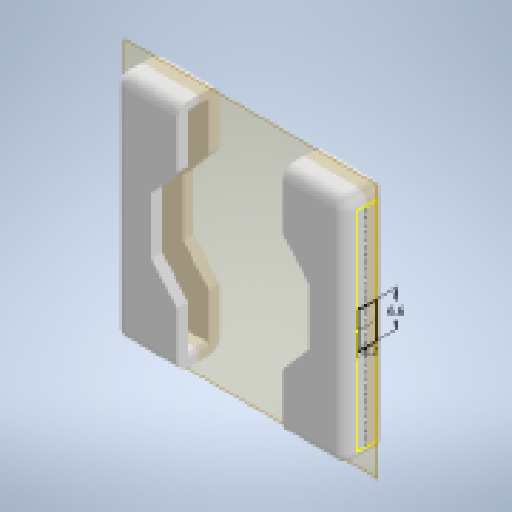
# Autodesk Inventor part: TurretCameraCover
Saved by Autodesk Inventor 2023 (Build 270158000, 158)
## iProperties
Created: 2023-05-07
Part Number: TurretCameraCover
Material: Generic
Document SubType Name: Modeling
Designer: karpova
Density: 1 g/cm^3
Appearance: Default
Author: karpova
Autodesk Inventor part; units mm, degrees
ref_plane "YZ Plane" through (0, 0, 0) normal (1, 0, 0) x (0, 1, 0)
ref_plane "XZ Plane" through (0, 0, 0) normal (0, 1, 0) x (-1, 0, 0)
sketch "Sketch1" plane through (0, 0, 0) normal (0, 0, 1) x (1, 0, 0)
  arc A0 (7.15, 17.4) -> (7.15, 16.1) centre (7.15, 16.75) ccw
  line L0 (7.15, 17.4) -> (17.4, 17.4)
  line L1 (17.4, 17.4) -> (17.4, 7.15)
  arc A1 (16.1, 7.15) -> (17.4, 7.15) centre (16.75, 7.15) ccw
  line L2 (16.1, 7.15) -> (16.1, 16.1)
  line L3 (16.1, 16.1) -> (7.15, 16.1)
  line L4 (-17.4, -17.4) -> (-17.4, -7.15)
  arc A2 (-16.1, -7.15) -> (-17.4, -7.15) centre (-16.75, -7.15) ccw
  line L5 (-16.1, -7.15) -> (-16.1, -16.1)
  line L6 (-16.1, -16.1) -> (-7.15, -16.1)
  arc A3 (-7.15, -17.4) -> (-7.15, -16.1) centre (-7.15, -16.75) ccw
  line L7 (-7.15, -17.4) -> (-17.4, -17.4)
  line L8 (3.95, -17.4) -> (-3.95, -17.4)
  arc A4 (-3.95, -16.1) -> (-3.95, -17.4) centre (-3.95, -16.75) ccw
  line L9 (-3.95, -16.1) -> (3.95, -16.1)
  arc A5 (3.95, -17.4) -> (3.95, -16.1) centre (3.95, -16.75) ccw
  line L10 (16.1, -16.1) -> (16.1, -7.15)
  arc A6 (17.4, -7.15) -> (16.1, -7.15) centre (16.75, -7.15) ccw
  line L11 (17.4, -7.15) -> (17.4, -17.4)
  line L12 (17.4, -17.4) -> (7.15, -17.4)
  arc A7 (7.15, -16.1) -> (7.15, -17.4) centre (7.15, -16.75) ccw
  line L13 (7.15, -16.1) -> (16.1, -16.1)
  line L14 (17.4, 3.95) -> (17.4, -3.95)
  arc A8 (16.1, -3.95) -> (17.4, -3.95) centre (16.75, -3.95) ccw
  line L15 (16.1, -3.95) -> (16.1, 3.95)
  arc A9 (17.4, 3.95) -> (16.1, 3.95) centre (16.75, 3.95) ccw
  line L16 (-17.4, -3.95) -> (-17.4, 3.95)
  arc A10 (-16.1, 3.95) -> (-17.4, 3.95) centre (-16.75, 3.95) ccw
  line L17 (-16.1, 3.95) -> (-16.1, -3.95)
  arc A11 (-17.4, -3.95) -> (-16.1, -3.95) centre (-16.75, -3.95) ccw
  circle A12 centre (-14.05, 14.05) radius 1.15
  circle A13 centre (14.05, 14.05) radius 1.15
  circle A14 centre (-14.05, -14.05) radius 1.15
  circle A15 centre (14.05, -14.05) radius 1.15
  arc A16 (-3.95, 17.4) -> (-3.95, 16.1) centre (-3.95, 16.75) ccw
  line L18 (-3.95, 17.4) -> (3.95, 17.4)
  arc A17 (3.95, 16.1) -> (3.95, 17.4) centre (3.95, 16.75) ccw
  line L19 (3.95, 16.1) -> (-3.95, 16.1)
  line L20 (-7.15, 16.1) -> (-16.1, 16.1)
  line L21 (-16.1, 16.1) -> (-16.1, 7.15)
  arc A18 (-17.4, 7.15) -> (-16.1, 7.15) centre (-16.75, 7.15) ccw
  line L22 (-17.4, 7.15) -> (-17.4, 17.4)
  line L23 (-17.4, 17.4) -> (-7.15, 17.4)
  arc A19 (-7.15, 16.1) -> (-7.15, 17.4) centre (-7.15, 16.75) ccw
  line L24 (19, -19) -> (19, 19)
  line L25 (19, 19) -> (-19, 19)
  line L26 (-19, 19) -> (-19, -19)
  line L27 (-19, -19) -> (19, -19)
  line L28 (-8, -2) -> (-9.776519, -2)
  arc A20 (-9.776519, 2) -> (-9.776519, -2) centre (-9.645728, 0) ccw
  line L29 (-9.776519, 2) -> (-8, 2)
  line L30 (-8, 2) -> (-8, 8)
  line L31 (-8, 8) -> (8, 8)
  line L32 (8, 8) -> (8, 2)
  line L33 (8, 2) -> (9.776519, 2)
  arc A21 (9.776519, -2) -> (9.776519, 2) centre (9.645728, 0) ccw
  line L34 (9.776519, -2) -> (8, -2)
  line L35 (8, -2) -> (8, -8)
  line L36 (8, -8) -> (-8, -8)
  line L37 (-8, -8) -> (-8, -2)
  line L38 (-19.1, 19.1) -> (19.1, 19.1)
  line L39 (19.1, 19.1) -> (19.1, -19.1)
  line L40 (19.1, -19.1) -> (-19.1, -19.1)
  line L41 (-19.1, -19.1) -> (-19.1, 19.1)
  line L42 (21.1, 21.1) -> (-21.1, 21.1)
  line L43 (-21.1, 21.1) -> (-21.1, -21.1)
  line L44 (-21.1, -21.1) -> (21.1, -21.1)
  line L45 (21.1, -21.1) -> (21.1, 21.1)
  line L46 (0, 21.1) -> (0, -21.1) construction
  line L47 (-9.645728, 21.1) -> (9.645728, 21.1)
  line L48 (9.645728, 21.1) -> (9.645728, -21.1)
  line L49 (9.645728, -21.1) -> (-9.645728, -21.1)
  line L50 (-9.645728, -21.1) -> (-9.645728, 21.1)
  point P0 (0, 0)
  point P1 (9.645728, -19.1)
  point P2 (9.645728, 19.1)
  point P3 (-9.645728, 19.1)
  point P4 (-9.645728, -19.1)
  dimension "d0" = 0.1
  dimension "d1" = 2
  constraints: 26 end point, 3 midpoint, 2 parallel, 2 point on line, 1 horizontal, 1 perpendicular, 7 other
  measures "d0" distance between parallel lines of L25 L38
  measures "d1" distance between parallel lines of L38 L42
ref_plane "Work Plane1" through (-19.052044, -19.052044, -1.6) normal (0, 0, -1) x (0, 1, 0)
extrude "Extrusion1" add sketch "Sketch1" against normal up to surface (1.6 mm away) contours L48 L42 L45 L44 L40 L39 L38 | L38 L41 L40 L50 L44 L43 L42
sketch "Sketch2" plane through (0, 0, 0) normal (0, 0, 1) x (1, 0, 0)
  line L0 (-19.1, 19.1) -> (-9.645728, 19.1)
  line L1 (-9.645728, 19.1) -> (-9.645728, 21.1)
  line L2 (-9.645728, 21.1) -> (-21.1, 21.1)
  line L3 (-21.1, 21.1) -> (-21.1, -21.1)
  line L4 (-21.1, -21.1) -> (-9.645728, -21.1)
  line L5 (-9.645728, -21.1) -> (-9.645728, -19.1)
  line L6 (-9.645728, -19.1) -> (-19.1, -19.1)
  line L7 (-19.1, -19.1) -> (-19.1, 19.1)
  line L8 (19.1, -19.1) -> (9.645728, -19.1)
  line L9 (9.645728, -19.1) -> (9.645728, -21.1)
  line L10 (9.645728, -21.1) -> (21.1, -21.1)
  line L11 (21.1, -21.1) -> (21.1, 21.1)
  line L12 (21.1, 21.1) -> (9.645728, 21.1)
  line L13 (9.645728, 21.1) -> (9.645728, 19.1)
  line L14 (9.645728, 19.1) -> (19.1, 19.1)
  line L15 (19.1, 19.1) -> (19.1, -19.1)
  point P0 (0, 0)
extrude "Extrusion2" add sketch "Sketch2" along normal blind 0.1
sketch "Sketch3" plane through (0, 0, 0.1) normal (0, 0, 1) x (1, 0, 0)
  line L0 (-9.645728, 19.1) -> (-9.645728, 21.1)
  line L1 (-9.645728, 21.1) -> (-21.1, 21.1)
  line L2 (-21.1, 21.1) -> (-21.1, -21.1)
  line L3 (-21.1, -21.1) -> (-9.645728, -21.1)
  line L4 (-9.645728, -21.1) -> (-9.645728, -19.1)
  line L5 (-9.645728, -19.1) -> (-19.1, -19.1)
  line L6 (-19.1, -19.1) -> (-19.1, 19.1)
  line L7 (-19.1, 19.1) -> (-9.645728, 19.1)
  line L8 (9.645728, -19.1) -> (9.645728, -21.1)
  line L9 (9.645728, -21.1) -> (21.1, -21.1)
  line L10 (21.1, -21.1) -> (21.1, 21.1)
  line L11 (21.1, 21.1) -> (9.645728, 21.1)
  line L12 (9.645728, 21.1) -> (9.645728, 19.1)
  line L13 (9.645728, 19.1) -> (19.1, 19.1)
  line L14 (19.1, 19.1) -> (19.1, -19.1)
  line L15 (19.1, -19.1) -> (9.645728, -19.1)
  line L16 (-21.1, 21.1) -> (-9.645728, 21.1)
  line L17 (-9.645728, -21.1) -> (-21.1, -21.1)
  line L18 (-21.1, -21.1) -> (-21.1, 21.1)
  line L19 (-9.645728, 10.807674) -> (-14.397033, 5.192326)
  line L20 (-14.397033, 5.192326) -> (-14.397033, -5.192326)
  line L21 (-14.397033, -5.192326) -> (-9.645728, -10.807674)
  line L22 (-9.645728, 21.1) -> (-9.645728, 10.807674)
  line L23 (-9.645728, -10.807674) -> (-9.645728, -21.1)
  line L24 (-21.1, 0) -> (-14.397033, 0) construction
  circle A0 centre (0, 0) radius 7.5 construction
  line L25 (-8, -8) -> (8, -8) construction
  line L26 (8, -8) -> (8, 8) construction
  line L27 (8, 8) -> (-8, 8) construction
  line L28 (-8, 8) -> (-8, -8) construction
  line L29 (-12.02138, -8) -> (8, -8) construction
  line L30 (-12.02138, 8) -> (8, 8) construction
  arc A1 (7.15, 17.4) -> (7.15, 16.1) centre (7.15, 16.75) ccw construction
  line L31 (7.15, 17.4) -> (17.4, 17.4) construction
  line L32 (17.4, 17.4) -> (17.4, 7.15) construction
  arc A2 (16.1, 7.15) -> (17.4, 7.15) centre (16.75, 7.15) ccw construction
  line L33 (16.1, 7.15) -> (16.1, 16.1) construction
  line L34 (16.1, 16.1) -> (7.15, 16.1) construction
  line L35 (-17.4, -17.4) -> (-17.4, -7.15) construction
  arc A3 (-16.1, -7.15) -> (-17.4, -7.15) centre (-16.75, -7.15) ccw construction
  line L36 (-16.1, -7.15) -> (-16.1, -16.1) construction
  line L37 (-16.1, -16.1) -> (-7.15, -16.1) construction
  arc A4 (-7.15, -17.4) -> (-7.15, -16.1) centre (-7.15, -16.75) ccw construction
  line L38 (-7.15, -17.4) -> (-17.4, -17.4) construction
  line L39 (3.95, -17.4) -> (-3.95, -17.4) construction
  arc A5 (-3.95, -16.1) -> (-3.95, -17.4) centre (-3.95, -16.75) ccw construction
  line L40 (-3.95, -16.1) -> (3.95, -16.1) construction
  arc A6 (3.95, -17.4) -> (3.95, -16.1) centre (3.95, -16.75) ccw construction
  line L41 (16.1, -16.1) -> (16.1, -7.15) construction
  arc A7 (17.4, -7.15) -> (16.1, -7.15) centre (16.75, -7.15) ccw construction
  line L42 (17.4, -7.15) -> (17.4, -17.4) construction
  line L43 (17.4, -17.4) -> (7.15, -17.4) construction
  arc A8 (7.15, -16.1) -> (7.15, -17.4) centre (7.15, -16.75) ccw construction
  line L44 (7.15, -16.1) -> (16.1, -16.1) construction
  line L45 (17.4, 3.95) -> (17.4, -3.95) construction
  arc A9 (16.1, -3.95) -> (17.4, -3.95) centre (16.75, -3.95) ccw construction
  line L46 (16.1, -3.95) -> (16.1, 3.95) construction
  arc A10 (17.4, 3.95) -> (16.1, 3.95) centre (16.75, 3.95) ccw construction
  line L47 (-17.4, -3.95) -> (-17.4, 3.95) construction
  arc A11 (-16.1, 3.95) -> (-17.4, 3.95) centre (-16.75, 3.95) ccw construction
  line L48 (-16.1, 3.95) -> (-16.1, -3.95) construction
  arc A12 (-17.4, -3.95) -> (-16.1, -3.95) centre (-16.75, -3.95) ccw construction
  circle A13 centre (-14.05, 14.05) radius 1.15 construction
  circle A14 centre (14.05, 14.05) radius 1.15 construction
  circle A15 centre (-14.05, -14.05) radius 1.15 construction
  circle A16 centre (14.05, -14.05) radius 1.15 construction
  arc A17 (-3.95, 17.4) -> (-3.95, 16.1) centre (-3.95, 16.75) ccw construction
  line L49 (-3.95, 17.4) -> (3.95, 17.4) construction
  arc A18 (3.95, 16.1) -> (3.95, 17.4) centre (3.95, 16.75) ccw construction
  line L50 (3.95, 16.1) -> (-3.95, 16.1) construction
  line L51 (-7.15, 16.1) -> (-16.1, 16.1) construction
  line L52 (-16.1, 16.1) -> (-16.1, 7.15) construction
  arc A19 (-17.4, 7.15) -> (-16.1, 7.15) centre (-16.75, 7.15) ccw construction
  line L53 (-17.4, 7.15) -> (-17.4, 17.4) construction
  line L54 (-17.4, 17.4) -> (-7.15, 17.4) construction
  arc A20 (-7.15, 16.1) -> (-7.15, 17.4) centre (-7.15, 16.75) ccw construction
  line L55 (19, -19) -> (19, 19) construction
  line L56 (19, 19) -> (-19, 19) construction
  line L57 (-19, 19) -> (-19, -19) construction
  line L58 (-19, -19) -> (19, -19) construction
  line L59 (-8, -2) -> (-9.776519, -2) construction
  arc A21 (-9.776519, 2) -> (-9.776519, -2) centre (-9.645728, 0) ccw construction
  line L60 (-9.776519, 2) -> (-8, 2) construction
  line L61 (-8, 2) -> (-8, 8) construction
  line L62 (-8, 8) -> (8, 8) construction
  line L63 (8, 8) -> (8, 2) construction
  line L64 (8, 2) -> (9.776519, 2) construction
  arc A22 (9.776519, -2) -> (9.776519, 2) centre (9.645728, 0) ccw construction
  line L65 (9.776519, -2) -> (8, -2) construction
  line L66 (8, -2) -> (8, -8) construction
  line L67 (8, -8) -> (-8, -8) construction
  line L68 (-8, -8) -> (-8, -2) construction
  line L69 (0, 19) -> (0, -19) construction
  line L70 (9.645728, 19.1) -> (9.645728, 21.1)
  line L71 (9.645728, 21.1) -> (21.1, 21.1)
  line L72 (21.1, 21.1) -> (21.1, -21.1)
  line L73 (21.1, -21.1) -> (9.645728, -21.1)
  line L74 (9.645728, -21.1) -> (9.645728, -19.1)
  line L75 (9.645728, -19.1) -> (19.1, -19.1)
  line L76 (19.1, -19.1) -> (19.1, 19.1)
  line L77 (19.1, 19.1) -> (9.645728, 19.1)
  line L78 (21.1, 21.1) -> (9.645728, 21.1)
  line L79 (9.645728, -21.1) -> (21.1, -21.1)
  line L80 (21.1, -21.1) -> (21.1, 21.1)
  line L81 (9.645728, 10.807674) -> (14.397033, 5.192326)
  line L82 (14.397033, 5.192326) -> (14.397033, -5.192326)
  line L83 (14.397033, -5.192326) -> (9.645728, -10.807674)
  line L84 (9.645728, 21.1) -> (9.645728, 10.807674)
  line L85 (9.645728, -10.807674) -> (9.645728, -21.1)
  line L86 (21.1, 0) -> (14.397033, 0) construction
  line L87 (17.4, -17.4) -> (17.4, -7.15) construction
  arc A23 (17.4, -7.15) -> (16.1, -7.15) centre (16.75, -7.15) ccw construction
  line L88 (16.1, -7.15) -> (16.1, -16.1) construction
  line L89 (17.4, -3.95) -> (17.4, 3.95) construction
  arc A24 (17.4, 3.95) -> (16.1, 3.95) centre (16.75, 3.95) ccw construction
  line L90 (16.1, 3.95) -> (16.1, -3.95) construction
  arc A25 (16.1, -3.95) -> (17.4, -3.95) centre (16.75, -3.95) ccw construction
  circle A26 centre (14.05, 14.05) radius 1.15 construction
  circle A27 centre (14.05, -14.05) radius 1.15 construction
  line L91 (16.1, 16.1) -> (16.1, 7.15) construction
  arc A28 (16.1, 7.15) -> (17.4, 7.15) centre (16.75, 7.15) ccw construction
  line L92 (17.4, 7.15) -> (17.4, 17.4) construction
  line L93 (19, 19) -> (19, -19) construction
  arc A29 (9.776519, -2) -> (9.776519, 2) centre (9.645728, 0) ccw construction
  point P0 (0, 0)
  point P1 (12.02138, -8)
  point P2 (12.02138, 8)
  constraints: 72 end point, 23 symmetric about line, 10 point on circle, 7 centre point, 6 midpoint, 5 collinear, 3 parallel, 2 equal length, 2 horizontal, 2 perpendicular, 1 vertical, 7 other
sketch "Sketch4" plane through (-9.645728, -21.1, -1.6) normal (0, 0, -1) x (-1, 0, 0)
  line L0 (-19.291456, 2) -> (-19.291456, 0)
  line L1 (-28.745728, 2) -> (-19.291456, 2)
  line L2 (-28.745728, 40.2) -> (-28.745728, 2)
  line L3 (-19.291456, 40.2) -> (-28.745728, 40.2)
  line L4 (-19.291456, 42.2) -> (-19.291456, 40.2)
  line L5 (-30.745728, 42.2) -> (-19.291456, 42.2)
  line L6 (-30.745728, 0) -> (-30.745728, 42.2)
  line L7 (-19.291456, 0) -> (-30.745728, 0)
  line L8 (0, 40.2) -> (0, 42.2)
  line L9 (9.454272, 40.2) -> (0, 40.2)
  line L10 (9.454272, 2) -> (9.454272, 40.2)
  line L11 (0, 2) -> (9.454272, 2)
  line L12 (0, 0) -> (0, 2)
  line L13 (11.454272, 0) -> (0, 0)
  line L14 (11.454272, 42.2) -> (11.454272, 0)
  line L15 (0, 42.2) -> (11.454272, 42.2)
  point P0 (-9.645728, 21.1)
extrude "Extrusion4" add sketch "Sketch4" along normal blind 2.1
ref_plane "Work Plane3" through (0, 0, -1.8) normal (0, 0, 1) x (1, 0, 0)
extrude "Extrusion5" add sketch "Sketch3" along normal blind 2
mirror "Mirror3" about plane through (0, 0, -1.8) normal (0, 0, 1) of "Extrusion5"
chamfer "Chamfer1" distance 0.5 angle 45 4 edges at (-9.6457, 19.1, -1.8) (9.6457, 19.1, -1.8) (9.6457, -19.1, -1.8) (-9.6457, -19.1, -1.8)
fillet "Fillet1" radius 2 16 edges at (-15.3729, -21.1, 2.1) (15.3729, -21.1, 2.1) (21.1, -21.1, -1.8) (-15.3729, 21.1, 2.1) (-21.1, 21.1, -1.8) (-15.3729, 21.1, -5.7) (15.3729, 21.1, -5.7) (21.1, 21.1, -1.8) (15.3729, 21.1, 2.1) (15.3729, -21.1, -5.7) (-15.3729, -21.1, -5.7) (-21.1, -21.1, -1.8) (21.1, 0, 2.1) (21.1, 0, -5.7) (-21.1, 0, 2.1) (-21.1, 0, -5.7)
sketch "Sketch7" plane through (14.397033, -5.192326, -5.7) normal (0, 0, -1) x (-1, 0, 0)
  line L0 (14.247033, -5.607674) -> (4.197033, -5.607674)
  line L1 (4.197033, -5.607674) -> (4.197033, -10.307674)
  line L2 (4.197033, -10.307674) -> (14.247033, -10.307674)
  line L3 (14.247033, -10.307674) -> (14.247033, -5.607674)
  line L4 (3.197033, -4.607674) -> (15.247033, -4.607674)
  line L5 (15.247033, -4.607674) -> (15.247033, -11.307674)
  line L6 (15.247033, -11.307674) -> (3.197033, -11.307674)
  line L7 (3.197033, -11.307674) -> (3.197033, -4.607674)
  line L8 (3.197033, -4.607674) -> (15.247033, -4.607674)
  line L9 (15.247033, -4.607674) -> (15.247033, -2.264195)
  line L10 (15.247033, -2.264195) -> (3.197033, -2.264195)
  line L11 (3.197033, -2.264195) -> (3.197033, -4.607674)
  point P0 (14.397033, 5.192326)
  point P1 (15.247033, -4.607674)
  dimension "d25" = 1
  constraints: 16 end point, 2 parallel, 1 horizontal, 1 perpendicular, 3 other
  measures "d25" distance between parallel lines of L0 L4
extrude "Extrusion8" cut sketch "Sketch7" against normal up to surface (2 mm away) contours L3 L2 L1 L0 | L11 L10 L9 L4 | L4 L5 L6 L7
sketch "Sketch8" plane through (21.1, -19.1, -3.7) normal (1, 0, 0) x (0, 0, -1)
  line L0 (0, 0) -> (-3.8, 0) projected
  line L1 (0, 38.2) -> (0, 0) projected
  line L2 (-3.8, 38.2) -> (0, 38.2) projected
  line L3 (-3.8, 0) -> (-3.8, 38.2) projected
  line L4 (-3.8, 38.2) -> (-3.8, 0) construction
  line L5 (-3.8, 19.1) -> (0, 19.1) construction
  line L6 (-3.5, 22.4) -> (-0.3, 22.4)
  line L7 (-0.3, 22.4) -> (-0.3, 15.8)
  line L8 (-0.3, 15.8) -> (-3.5, 15.8)
  line L9 (-3.5, 15.8) -> (-3.5, 22.4)
  line L10 (-1.9, 38.2) -> (-1.9, 0) construction
  point P0 (-3.7, 19.1)
  dimension "d28" = 3.2
  dimension "d29" = 6.6
  constraints: 12 end point, 4 midpoint, 2 parallel, 1 horizontal, 1 perpendicular, 2 other
  measures "d28" distance of L7.end L8.end
  measures "d29" distance of L6.end L7.end
extrude "Extrusion9" add sketch "Sketch8" along normal blind 3 contours L6 L7 L8 L9
sketch "Sketch9" plane through (-21.1, -19.1, 0.1) normal (-1, 0, 0) x (0, 0, 1)
  line L0 (-0.3, 15.8) -> (-3.5, 15.8) projected
  line L1 (-3.5, 15.8) -> (-3.5, 22.4) projected
  line L2 (-3.5, 22.4) -> (-0.3, 22.4) projected
  line L3 (-0.3, 22.4) -> (-0.3, 15.8) projected
  point P0 (-0.1, 19.1)
extrude "Extrusion10" add sketch "Sketch9" along normal blind 3
body "Solid1"
